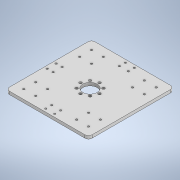
# Autodesk Inventor part: 升降板
Saved by Autodesk Inventor 2021 (Build 250183000, 183)
## iProperties
Created: 2023-02-14
Part Number: 升降板
Material: 一般
Document SubType Name: Sheet Metal
Designer: brian
Density: 1 g/cm^3
Sheet Metal Rule: 預設 mm (_M)
Appearance: 預設
Flat Pattern Width: 13.9 cm
Flat Pattern Length: 14.4 cm
Flat Pattern Area: 200.16 cm^2
Sheet Metal Width: 139.000 mm
Sheet Metal Length: 144.000 mm
Sheet Metal Area: 20016.000 mm^2
Author: brian
Autodesk Inventor part; units mm, degrees
ref_plane "YZ Plane" through (0, 0, 0) normal (1, 0, 0) x (0, 1, 0)
ref_plane "XZ Plane" through (0, 0, 0) normal (0, 1, 0) x (-1, 0, 0)
ref_plane "XY Plane" through (0, 0, 0) normal (0, 0, 1) x (1, 0, 0)
sketch "草圖1" plane through (0, 0, 0) normal (0, 1, 0) x (-1, 0, 0)
  line L0 (-69.5, 72) -> (69.5, 72)
  line L1 (69.5, 72) -> (69.5, -72)
  line L2 (69.5, -72) -> (-69.5, -72)
  line L3 (-69.5, -72) -> (-69.5, 72)
  line L4 (-69.5, 72) -> (69.5, -72) construction
  line L5 (69.5, 72) -> (-69.5, -72) construction
  point P0 (0, 0)
  dimension "d0" = 139
  dimension "d1" = 144
  measures "d0" distance of L1.end L2.end
  measures "d1" distance of L0.end L1.end
extrude "平板1" add sketch "草圖1" along normal blind 5
sketch "草圖2" plane through (0, 5, 0) normal (0, 1, 0) x (1, 0, 0)
  circle A0 centre (0, 0) radius 12.1
  dimension "d4" = 24.2
  constraints: 1 centre point, 1 coincident
  measures "d4" diameter of A0
extrude "切割1" cut sketch "草圖2" against normal blind 5
sketch "草圖3" plane through (0, 5, 0) normal (0, 1, 0) x (1, 0, 0)
  point P0 (0, 0)
  point P1 (0, -16)
  dimension "d7" = 16
  constraints: 1 vertical alignment
  measures "d7" distance of point (0, -16) point (0, 0)
hole "孔1" at (0, 5, 16) direction (0, -1, 0) diameter 4.5 end through all
pattern_circular "環形陣列1" count 8 over 360 about axis through (0, 5, 0) along (0, -1, 0) of "孔1"
sketch "草圖4" plane through (0, 5, 0) normal (0, 1, 0) x (1, 0, 0)
  line L0 (69.5, -72) -> (-69.5, -72) projected
  point P0 (0, 0)
  point P1 (-7.5, -67)
  point P2 (-7.5, -57)
  point P3 (7.5, -67)
  point P4 (7.5, -57)
  point P5 (63.5, -72)
  point P6 (-63.5, -72)
  dimension "d18" = 10
  dimension "d19" = 15
  dimension "d20" = 5
  dimension "d21" = 7.5
  constraints: 2 horizontal alignment, 2 vertical alignment
  measures "d18" distance of point (-7.5, -57) point (-7.5, -67)
  measures "d19" distance of point (7.5, -67) point (-7.5, -67)
  measures "d20" distance from line of L0 point (7.5, -67)
  measures "d21" horizontal distance of point (0, 0) point (-7.5, -67)
hole "孔2" at (-7.5, 5, 67) at (-7.5, 5, 57) at (7.5, 5, 67) at (7.5, 5, 57) direction (0, -1, 0) diameter 3.1 end through all
sketch "草圖5" plane through (0, 5, 0) normal (0, 1, 0) x (1, 0, 0)
  line L0 (-64.5, -7.5) -> (-54.5, -7.5)
  line L1 (-54.5, -7.5) -> (-54.5, 7.5)
  line L2 (-54.5, 7.5) -> (-64.5, 7.5)
  line L3 (-64.5, 7.5) -> (-64.5, -7.5)
  line L4 (-69.5, -72) -> (-69.5, 72) projected
  point P0 (0, 0)
  point P1 (-69.5, -66)
  point P2 (-69.5, 66)
  point P3 (-54.5, 0)
  dimension "d29" = 15
  dimension "d30" = 10
  dimension "d31" = 5
  constraints: 8 end point, 4 coincident, 2 parallel, 1 horizontal, 1 horizontal alignment, 1 midpoint, 1 perpendicular
  measures "d29" distance of L0.end L1.end
  measures "d30" distance of L1.end L2.end
  measures "d31" distance between parallel lines of L4 L3
hole "孔3" at (-64.5, 5, 7.5) at (-64.5, 5, -7.5) at (-54.5, 5, -7.5) at (-54.5, 5, 7.5) direction (0, -1, 0) diameter 3.1 end through all
mirror "鏡射1" about plane through (0, 0, 0) normal (0, 0, 1) of "孔2"
sketch "草圖7" plane through (0, 5, 0) normal (0, 1, 0) x (1, 0, 0)
  line L0 (-54.5, -57) -> (-34.5, -57)
  line L1 (-34.5, -57) -> (-34.5, -37)
  line L2 (-34.5, -37) -> (-54.5, -37)
  line L3 (-54.5, -37) -> (-54.5, -57)
  line L4 (-69.5, -72) -> (-69.5, 72) projected
  line L5 (69.5, -72) -> (-69.5, -72) projected
  point P0 (0, 0)
  dimension "d53" = 20
  dimension "d54" = 20
  dimension "d64" = 15
  dimension "d65" = 15
  constraints: 8 end point, 4 coincident, 2 parallel, 1 horizontal, 1 perpendicular
  measures "d53" distance of L2.end L1.end
  measures "d54" distance of L1.end L0.end
  measures "d64" distance between parallel lines of L5 L0
  measures "d65" distance between parallel lines of L4 L3
hole "孔4" at (-54.5, 5, 57) at (-34.5, 5, 57) at (-34.5, 5, 37) at (-54.5, 5, 37) direction (0, -1, 0) diameter 3.2 end through all
mirror "鏡射2" about plane through (0, 0, 0) normal (0, 0, 1) of "孔4"
mirror "鏡射3" about plane through (0, 0, 0) normal (1, 0, 0) of "孔4", "鏡射2"
fillet "轉角外圓角2" radius 6 4 edges at (69.5, 2.5, 72) (69.5, 2.5, -72) (-69.5, 2.5, -72) (-69.5, 2.5, 72)
sketch "草圖6" plane through (70.5, 6, -72) normal (1, 0, 0) x (0, 1, 0)
  line L0 (0, 144) -> (0, 0)
  line L1 (0, 0) -> (4, 0)
  line L2 (4, 0) -> (4, 144)
  line L3 (4, 144) -> (0, 144)
  constraints: 6 end point, 1 horizontal, 1 perpendicular, 1 vertical
equation "\"d5\" = 厚度"
equation "\"d13\" = 厚度"
equation "\"d21\" = 0.5 * d19"
equation "\"d27\" = 厚度"
equation "\"d29\" = d19"
equation "\"d30\" = d18"
equation "\"d31\" = d20"
equation "\"d32\" = d22"
equation "\"d37\" = 厚度"
equation "\"d54\" = d53"
equation "\"d62\" = 厚度"
equation "\"d2\" = 厚度"
equation "\"折彎半徑\" = 厚度"
equation "\"折彎離隙寬度\" = 厚度"
equation "\"折彎離隙深度\" = 0.5 * 厚度"
equation "\"轉移半徑\" = 折彎半徑"
equation "\"Jacobi半徑大小\" = 折彎半徑"
equation "\"間隙大小\" = 厚度"
equation "\"厚度\" = 5"
equation "\"d22\" = 3.1"
